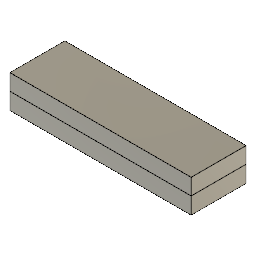
Display-MAX7219-LED-Esphome (Autodesk Fusion 360 design; units mm, degrees)
Autodesk Fusion 360 part; units mm, degrees
sketch "Esquisse1" plane through (0, 0, 0) normal (0, 0, 1) x (1, 0, 0)
  line L0 (0, 0) -> (135, 0)
  line L1 (135, 0) -> (135, 41)
  line L2 (135, 41) -> (0, 41)
  line L3 (0, 41) -> (0, 0)
  dimension "d1" = 135
  dimension "d2" = 41
  constraint horizontal L0
  constraint vertical L1
  constraint horizontal L2
  constraint vertical L3
  constraint coincident L0.start L3.end
  measures "d1" distance of L0.start L0.end
  measures "d2" distance of L0.start L2.end
extrude "Extrusion3" add sketch "Esquisse1" along normal blind 0.48 makes body 1
sketch "Esquisse3" plane through (0, 0, 0.48) normal (0, 0, 1) x (-1, 0, 0)
  line L0 (0, -41) -> (0, 0)
  line L1 (0, 0) -> (-135, 0)
  line L2 (-135, 0) -> (-135, -41)
  line L3 (-135, -41) -> (0, -41)
  line L4 (-2, -2) -> (-133, -2)
  line L5 (-133, -2) -> (-133, -39)
  line L6 (-133, -39) -> (-2, -39)
  line L7 (-2, -39) -> (-2, -2)
  dimension "d11" = -2
extrude "Extrusion5" add sketch "Esquisse3" along normal blind 14 bodies 1
sketch "Esquisse4" plane through (0, 0, 14.48) normal (0, 0, 1) x (-1, 0, 0)
  line L0 (-2, -2) -> (-2, -39)
  line L1 (-2, -39) -> (-133, -39)
  line L2 (-133, -39) -> (-133, -2)
  line L3 (-133, -2) -> (-2, -2)
  line L4 (-135, -41) -> (0, -41)
  line L5 (0, -41) -> (0, 0)
  line L6 (0, 0) -> (-135, 0)
  line L7 (-135, 0) -> (-135, -41)
  line L8 (-1, -1) -> (-134, -1)
  line L9 (-134, -1) -> (-134, -40)
  line L10 (-134, -40) -> (-1, -40)
  line L11 (-1, -40) -> (-1, -1)
  dimension "d14" = -1
extrude "Extrusion6" cut sketch "Esquisse4" against normal blind 2 contours L4 L5 L6 L7 bodies 1
sketch "Esquisse4 (2)" plane through (0, 0, 12.48) normal (0, 0, 1) x (-1, 0, 0) in component "Couvercle"
  line L0 (-1, -1) -> (-1, -40)
  line L1 (-1, -40) -> (-134, -40)
  line L2 (-134, -40) -> (-134, -1)
  line L3 (-134, -1) -> (-1, -1)
  line L4 (-135, 0) -> (-135, -41)
  line L5 (-135, -41) -> (0, -41)
  line L6 (0, -41) -> (0, 0)
  line L7 (0, 0) -> (-135, 0)
  line L8 (0, 0) -> (-135, 0)
  line L9 (-135, 0) -> (-135, -41)
  line L10 (-135, -41) -> (0, -41)
  line L11 (0, -41) -> (0, 0)
  line L12 (-134.05, -40.05) -> (-0.95, -40.05)
  line L13 (-0.95, -40.05) -> (-0.95, -0.95)
  line L14 (-0.95, -0.95) -> (-134.05, -0.95)
  line L15 (-134.05, -0.95) -> (-134.05, -40.05)
  dimension "d28" = -0.95
  constraint horizontal L8
  constraint vertical L9
  constraint horizontal L10
  constraint vertical L11
  constraint coincident L4.end L5.start
  constraint coincident L6.end L7.start
extrude "Extrusion1" add sketch "Esquisse4 (2)" along normal blind 10 separate body contours L4 L5 L6 L7 L8 L9 L10 L11 makes body 2 in component "Couvercle"
sketch "Esquisse5" plane through (0, 0, 22.48) normal (0, 0, 1) x (-1, 0, 0) in component "Couvercle"
  line L0 (-134.05, -40.05) -> (-134.05, -0.95)
  line L1 (-134.05, -0.95) -> (-0.95, -0.95)
  line L2 (-0.95, -0.95) -> (-0.95, -40.05)
  line L3 (-0.95, -40.05) -> (-134.05, -40.05)
  line L4 (0, -41) -> (0, 0)
  line L5 (0, 0) -> (-135, 0)
  line L6 (-135, 0) -> (-135, -41)
  line L7 (-135, -41) -> (0, -41)
  line L8 (0, 0) -> (-135, 0)
  line L9 (-135, 0) -> (-135, -41)
  line L10 (-135, -41) -> (0, -41)
  line L11 (0, -41) -> (0, 0)
  constraint horizontal L8
  constraint vertical L9
  constraint horizontal L10
  constraint vertical L11
  constraint coincident L6.end L7.start
  constraint coincident L4.end L5.start
extrude "Extrusion2" add sketch "Esquisse5" along normal blind 2 contours L0 L1 L2 L3 | L4 L5 L6 L7 L8 L9 L10 L11 bodies 2 in component "Couvercle"
sketch "Esquisse7" plane through (0, 0, 22.48) normal (0, 0, -1) x (1, 0, 0) in component "Couvercle"
  line L0 (0.95, -40.05) -> (134.05, -40.05)
  line L1 (134.05, -40.05) -> (134.05, -0.95)
  line L2 (134.05, -0.95) -> (0.95, -0.95)
  line L3 (0.95, -0.95) -> (0.95, -40.05)
  line L4 (0.95, -33.55) -> (35.95, -33.55)
  line L5 (35.95, -33.55) -> (35.95, -7.55)
  line L6 (35.95, -7.55) -> (0.95, -7.55)
  line L7 (0.95, -7.55) -> (0.95, -33.55)
  line L8 (0.95, -35.55) -> (37.95, -35.55)
  line L9 (37.95, -35.55) -> (37.95, -5.55)
  line L10 (37.95, -5.55) -> (0.95, -5.55)
  dimension "d33" = 35
  dimension "d34" = 26
  dimension "d35" = 6.6
  constraint horizontal L4
  constraint vertical L5
  constraint horizontal L6
  constraint vertical L7
  constraint coincident L3 L4.start
  constraint coincident L3 L8.start
  constraint coincident L3 L10.end
  measures "d33" distance of L4.start L4.end
  measures "d34" distance of L4.start L6.end
  measures "d35" distance of L2 L6
extrude "Extrusion3'" add sketch "Esquisse7" along normal blind 7 contours L3 L4 L5 L6 L8 L9 L10 bodies 2 in component "Couvercle"
sketch "Esquisse8" plane through (0, 0, 0) normal (-1, 0, 0) x (0, -1, 0) in component "Couvercle"
  line L0 (-41, 12.48) -> (0, 12.48)
  line L1 (0, 12.48) -> (0, 24.48)
  line L2 (0, 24.48) -> (-41, 24.48)
  line L3 (-41, 24.48) -> (-41, 12.48)
  line L4 (-25.5, 21) -> (-15.5, 21)
  line L5 (-15.5, 21) -> (-15.5, 17)
  line L6 (-15.5, 17) -> (-25.5, 17)
  line L7 (-25.5, 17) -> (-25.5, 21)
  line L8 (-26.5, 23) -> (-14.5, 23)
  line L9 (-14.5, 23) -> (-14.5, 15)
  line L10 (-14.5, 15) -> (-26.5, 15)
  line L11 (-26.5, 15) -> (-26.5, 23)
  dimension "d39" = 10
  dimension "d40" = 4
  dimension "d41" = 21
  dimension "d42" = 15.5
  dimension "d43" = 12
  dimension "d44" = 8
  dimension "d45" = 1
  dimension "d46" = 2
  constraint horizontal L4
  constraint vertical L5
  constraint horizontal L6
  constraint vertical L7
  constraint horizontal L8
  constraint vertical L9
  constraint horizontal L10
  constraint vertical L11
  measures "d39" distance of L4.start L4.end
  measures "d40" distance of L4.start L6.end
  measures "d41" distance of origin L4
  measures "d42" distance of L1 L5
  measures "d43" distance of L8.start L8.end
  measures "d44" distance of L8.start L10.end
  measures "d45" distance of L7 L11
  measures "d46" distance of L4 L8
extrude "Extrusion4" cut sketch "Esquisse8" against normal up to surface (0.95 mm away) contours L4 L5 L6 L7 bodies 2 in component "Couvercle"
extrude "Extrusion5'" cut sketch "Esquisse8" against normal blind 0.5 contours L8 L9 L10 L11 bodies 2 in component "Couvercle"
fillet "Congé1" radius 0.3 1 edges at (134.05, 40.05, 17.48) on bodies 2 in component "Couvercle"
extrude "Extrusion6'" add 1 faces at (24.2833, 16.2167, 22.48) along direction (0, 0, -1) blind 0.5 on bodies 2 bodies 2 in component "Couvercle"
sketch "Esquisse9" plane through (0, 0, 15.48) normal (0, 0, -1) x (1, 0, 0) in component "Couvercle"
  line L0 (0.95, -33.55) -> (0.95, -35.55)
  line L1 (0.95, -35.55) -> (37.95, -35.55)
  line L2 (37.95, -35.55) -> (37.95, -5.55)
  line L3 (37.95, -5.55) -> (0.95, -5.55)
  line L4 (0.95, -5.55) -> (0.95, -7.55)
  line L5 (0.95, -7.55) -> (35.95, -7.55)
  line L6 (35.95, -7.55) -> (35.95, -33.55)
  line L7 (35.95, -33.55) -> (0.95, -33.55)
  line L8 (35.95, -20.55) -> (35.95, -18.05)
  line L9 (37.95, -18.05) -> (37.95, -23.05)
  line L10 (35.95, -18.05) -> (37.95, -18.05)
  line L11 (37.95, -23.05) -> (35.95, -23.05)
  line L12 (35.95, -20.55) -> (35.95, -18.05)
  line L13 (35.95, -23.05) -> (35.95, -20.55)
  dimension "d58" = 2.5
  dimension "d59" = 5
  constraint midpoint L6 L8.start
  constraint coincident L6 L8.end
  constraint coincident L2 L9.start
  constraint parallel L2 L9
  constraint perpendicular L9 L10
  constraint coincident L6 L11.end
  constraint perpendicular L6 L11
  measures "d58" distance of L8.start L8.end
  measures "d59" distance of L9.start L9.end
extrude "Extrusion7" cut sketch "Esquisse9" against normal up to surface (7 mm away) contours L2 L6 L8 L9 L10 L11 L12 L13 bodies 2 in component "Couvercle"
sketch "Esquisse10" plane through (0, 0, 22.48) normal (0, 0, -1) x (1, 0, 0) in component "Couvercle"
  arc A0 (133.75, -40.05) -> (134.05, -39.75) centre (133.75, -39.75) ccw
  line L0 (134.05, -39.75) -> (134.05, -0.95)
  line L1 (134.05, -0.95) -> (0.95, -0.95)
  line L2 (0.95, -0.95) -> (0.95, -5.55)
  line L3 (0.95, -5.55) -> (37.95, -5.55)
  line L4 (37.95, -5.55) -> (37.95, -18.05)
  line L5 (37.95, -18.05) -> (35.95, -18.05)
  line L6 (35.95, -18.05) -> (35.95, -23.05)
  line L7 (35.95, -23.05) -> (37.95, -23.05)
  line L8 (37.95, -23.05) -> (37.95, -35.55)
  line L9 (37.95, -35.55) -> (0.95, -35.55)
  line L10 (0.95, -35.55) -> (0.95, -40.05)
  line L11 (0.95, -40.05) -> (133.75, -40.05)
  circle A1 centre (115, -18.25) radius 5
  circle A2 centre (80, -18.25) radius 5
  circle A3 centre (50, -18.25) radius 5
  line L12 (135, 0) -> (135, -41)
  dimension "d62" = 10
  dimension "d63" = 10
  dimension "d66" = 10
  dimension "d67" = 20
  dimension "d70" = 35
  dimension "d71" = 30
  measures "d62" diameter of A1
  measures "d63" diameter of A2
  measures "d66" diameter of A3
  measures "d67" distance of A1.centre L12
  measures "d70" distance of A1.centre A2.centre
  measures "d71" distance of A2.centre A3.centre
extrude "Extrusion8" add sketch "Esquisse10" along normal blind 7 contours A1 | A2 | A3 bodies 2 in component "Couvercle"
sketch "Esquisse11" plane through (0, 0, 21.98) normal (0, 0, -1) x (1, 0, 0) in component "Couvercle"
  line L0 (35.95, -7.55) -> (0.95, -7.55)
  line L1 (0.95, -7.55) -> (0.95, -33.55)
  line L2 (0.95, -33.55) -> (35.95, -33.55)
  line L3 (35.95, -33.55) -> (35.95, -23.05)
  line L4 (35.95, -23.05) -> (35.95, -18.05)
  line L5 (35.95, -18.05) -> (35.95, -7.55)
  line L6 (35.95, -7.55) -> (20.95, -7.55)
  line L7 (20.95, -7.55) -> (20.95, -10.55)
  line L8 (20.95, -10.55) -> (35.95, -10.55)
  line L9 (35.95, -10.55) -> (35.95, -7.55)
  line L10 (35.95, -33.55) -> (20.95, -33.55)
  line L11 (20.95, -33.55) -> (20.95, -30.55)
  line L12 (20.95, -30.55) -> (35.95, -30.55)
  line L13 (35.95, -30.55) -> (35.95, -33.55)
  line L14 (1.5462, -20.5) -> (1.5462, -15.5)
  line L15 (1.5462, -20.5) -> (1.5462, -25.5)
  line L16 (1.5462, -15.5) -> (6.5462, -15.5)
  line L17 (1.5462, -25.5) -> (6.5462, -25.5)
  line L18 (6.5462, -25.5) -> (6.5462, -15.5)
  dimension "d72" = 15
  dimension "d73" = 3
  dimension "d76" = 15
  dimension "d77" = 3
  dimension "d78" = 5
  dimension "d79" = 5
  dimension "d80" = 5
  dimension "d81" = 5
  constraint horizontal L6
  constraint vertical L7
  constraint horizontal L8
  constraint vertical L9
  constraint coincident L0.start L5.end
  constraint horizontal L10
  constraint vertical L11
  constraint horizontal L12
  constraint vertical L13
  constraint coincident L2.end L3.start
  constraint parallel L1 L14
  constraint parallel L1 L15
  constraint perpendicular L14 L16
  constraint perpendicular L15 L17
  measures "d72" distance of L0.start L6.end
  measures "d73" distance of L0.start L8.end
  measures "d76" distance of L2.end L10.end
  measures "d77" distance of L2.end L12.end
  measures "d78" distance of L14.start L14.end
  measures "d79" distance of L14.start L15.end
  measures "d80" distance of L14.end L16.end
  measures "d81" distance of L15.end L17.end
extrude "Extrusion9" add sketch "Esquisse11" along normal blind 3 contours L0 L5 L6 L7 L8 L9 bodies 2 in component "Couvercle"
extrude "Extrusion10" add sketch "Esquisse11" along normal blind 1 contours L14 L15 L16 L17 L18 bodies 2 in component "Couvercle"
extrude "Extrusion11" add sketch "Esquisse11" along normal blind 1 contours L2 L3 L10 L11 L12 L13 bodies 2 in component "Couvercle"
sketch "Esquisse5 (2)" plane through (0, 0, 0.48) normal (0, 0, 1) x (-1, 0, 0)
  line L0 (-2, -2) -> (-133, -2)
  line L1 (-133, -2) -> (-133, -39)
  line L2 (-133, -39) -> (-2, -39)
  line L3 (-2, -39) -> (-2, -2)
  line L4 (-2, -39) -> (-133, -39)
  line L5 (-133, -39) -> (-133, -36)
  line L6 (-133, -36) -> (-2, -36)
  line L7 (-2, -36) -> (-2, -39)
  dimension "d47" = 3
  constraint horizontal L4
  constraint vertical L5
  constraint horizontal L6
  constraint vertical L7
  constraint coincident L2.end L3.start
  measures "d47" distance of L2.end L6.end
extrude "Extrusion7'" [suppressed]
component "Couvercle" placed x (1, 0, 0) y (0, 1, 0) z (0, 0, 1) at (0, 0, 0)
named bodies: "Socle"
